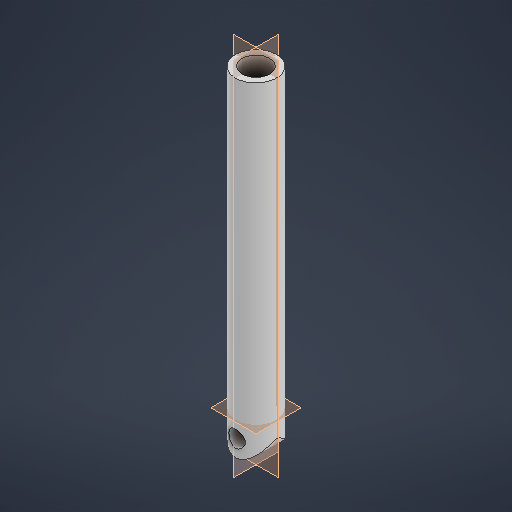
# Autodesk Inventor part: Cylinder_Bom
Saved by Autodesk Inventor 2026 (Build 300175000, 175)
## iProperties
Created: 2025-05-02
Part Number: Cylinder_Bom
Material: Generic
Document SubType Name: Modeling
Designer: elias
Density: 1 g/cm^3
Appearance: Default
Author: elias
Autodesk Inventor part; units mm, degrees
sketch "Sketch1" plane through (0, 0, 0) normal (0, 1, 0) x (-1, 0, 0)
  circle A0 centre (0, 0) radius 37.5
  circle A1 centre (0, 0) radius 25
  dimension "d0" = 75
  dimension "d1" = 50
  constraints: 2 centre point, 2 coincident
  measures "d0" diameter of A0
  measures "d1" diameter of A1
extrude "Extrusion1" add sketch "Sketch1" along normal blind 540
sketch "Sketch2" plane through (0, 0, 0) normal (0, 1, 0) x (-1, 0, 0)
  line L0 (-37.5, -37.5) -> (37.5, -37.5)
  line L1 (37.5, -37.5) -> (37.5, 37.5)
  line L2 (37.5, 37.5) -> (-37.5, 37.5)
  line L3 (-37.5, 37.5) -> (-37.5, -37.5)
  point P0 (0, 0)
  constraints: 8 end point, 2 parallel, 1 horizontal, 1 perpendicular
extrude "Extrusion2" add sketch "Sketch2" against normal blind 60
sketch "Sketch3" plane through (0, 0, 0) normal (0, 0, 1) x (1, 0, 0)
  circle A0 centre (0, -30) radius 15
  line L0 (-52.5, 0) -> (52.5, 0) projected
  line L1 (-37.5, 0) -> (-37.5, -60) projected
  line L2 (37.5, 0) -> (37.5, -60) projected
  arc A1 (-37.5, -30) -> (37.5, -30) centre (0, -21.5625) ccw
  line L3 (-37.5, -30) -> (-52.5, -30)
  line L4 (-52.5, -30) -> (-52.5, -80.2965)
  line L5 (-52.5, -80.2965) -> (57.4115, -80.2965)
  line L6 (57.4115, -80.2965) -> (57.4115, -30)
  line L7 (57.4115, -30) -> (37.5, -30)
  point P0 (0, 0)
  dimension "d6" = 30
  dimension "d7" = 30
  constraints: 10 end point, 4 perpendicular, 2 centre point, 2 midpoint, 2 point on circle, 1 horizontal, 1 point on line
  measures "d6" diameter of A0
  measures "d7" distance from line of L0 A0.centre
extrude "Extrusion3" cut sketch "Sketch3" along normal mid plane 150 contours A0 | A1 L7 L6 L5 L4 L3
fillet "Fillet1" radius 37.5 4 edges at (37.5, -15, 37.5) (37.5, -15, -37.5) (-37.5, -15, 37.5) (-37.5, -15, -37.5)
body "Solid1"
